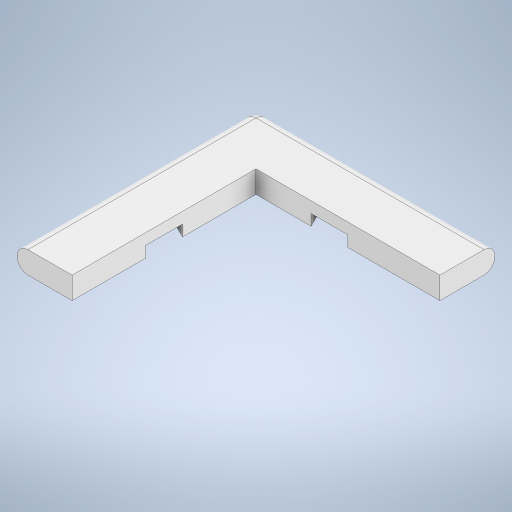
# Autodesk Inventor part: Test2
Saved by Autodesk Inventor 2023.1 (Build 271208000, 208)
## iProperties
Created: 2023-02-07
Part Number: Test2
Material: ABS Plastic
Document SubType Name: Modeling
Designer: 19644
Density: 1.06 g/cm^3
Appearance: Smooth - White
Author: 19644
## iProperties of the stored document Test2_3DPrint.ipt
Created: 2023-02-07
Part Number: Test2_3DPrint
Material: Generic
Document SubType Name: Modeling
Designer: 19644
Density: 1 g/cm^3
Appearance: Default
Author: 19644
Autodesk Inventor part; units mm, degrees
ref_plane "YZ Plane" through (0, 0, 0) normal (1, 0, 0) x (0, 1, 0)
ref_plane "XZ Plane" through (0, 0, 0) normal (0, 1, 0) x (-1, 0, 0)
ref_plane "XY Plane" through (0, 0, 0) normal (0, 0, 1) x (1, 0, 0)
sketch "Sketch1" plane through (0, 0, 0) normal (0, 1, 0) x (-1, 0, 0)
  line L0 (100, -50) -> (-100, -50)
  line L1 (-100, -50) -> (-100, 50)
  line L2 (100, -50) -> (-100, 50) construction
  line L3 (-100, -50) -> (100, 50) construction
  line L4 (-40, -30) -> (-80, -30)
  line L5 (-50, -50) -> (-70, -50)
  line L6 (-40, -30) -> (-50, -50)
  line L7 (-80, -30) -> (-70, -50)
  line L8 (70, -50) -> (50, -50)
  line L9 (-100, -10) -> (-100, 10)
  line L10 (-80, -20) -> (-80, 20)
  line L11 (-80, -20) -> (-100, -10)
  line L12 (-80, 20) -> (-100, 10)
  line L13 (-100, -50) -> (-130, -50)
  line L14 (-130, -50) -> (-130, 50)
  line L15 (-130, 50) -> (-100, 50)
  line L16 (-100, 50) -> (-100, -50)
  line L17 (-130, -50) -> (0, -50)
  line L18 (0, -50) -> (0, -80)
  line L19 (0, -80) -> (-130, -80)
  line L20 (-130, -80) -> (-130, -50)
  line L21 (-40, -70) -> (-80, -70)
  line L22 (-40, -70) -> (-50, -50)
  line L23 (-80, -70) -> (-70, -50)
  line L24 (-120, -20) -> (-120, 20)
  line L25 (-120, -20) -> (-100, -10)
  line L26 (-120, 20) -> (-100, 10)
  line L27 (40, -70) -> (50, -50)
  line L28 (40, -70) -> (80, -70)
  line L29 (80, -70) -> (70, -50)
  line L30 (100, -50) -> (100, 50)
  line L31 (130, -50) -> (130, 50)
  line L32 (130, 50) -> (100, 50)
  line L33 (130, -50) -> (0, -50)
  line L34 (0, -80) -> (130, -80)
  line L35 (130, -80) -> (130, -50)
  line L36 (40, -70) -> (50, -50)
  line L37 (40, -70) -> (80, -70)
  line L38 (80, -70) -> (70, -50)
  line L39 (120, -20) -> (100, -10)
  line L40 (120, 20) -> (100, 10)
  line L41 (120, -20) -> (120, 20)
  point P0 (0, 0)
  point P1 (-100, 10)
  point P2 (-100, -10)
  point P3 (-70, -50)
  point P4 (-50, -50)
  point P5 (0, 0)
  point P6 (0, 0)
  point P7 (0, -50)
  dimension "d72" = 200
  dimension "d73" = 100
  dimension "d78" = 20
  dimension "d79" = 40
  dimension "d80" = 20
  dimension "d81" = 10
  dimension "d82" = 20
  dimension "d86" = 120
  dimension "d88" = 0
  dimension "d90" = 40
  dimension "d91" = 20
  dimension "d92" = 20
  dimension "d93" = 10
  dimension "d94" = 40
  dimension "d95" = 0
  dimension "d114" = 30
  dimension "d115" = 130
  dimension "d116" = 30
  constraints: 84 end point, 15 symmetric about line, 6 horizontal, 4 parallel, 3 midpoint, 3 perpendicular, 2 vertical, 1 coincident
  measures "d72" distance of L1.end L3.end
  measures "d73" distance of L0.end L1.end
  measures "d78" distance of L5.start L5.end
  measures "d79" distance of L4.start L4.end
  measures "d80" distance from line of L5.end L4
  measures "d81" horizontal distance of L4.end L5.end
  measures "d82" distance of L8.start L8.end
  measures "d86" distance of L5.end L8.end
  measures "d88" distance between parallel lines of L0 L5
  measures "d90" distance of L10.start L10.end
  measures "d91" distance of L9.start L9.end
  measures "d92" distance between parallel lines of L9 L10
  measures "d93" vertical distance of L10.start L9.start
  measures "d94" distance from line of L0 L9.start
  measures "d95" distance between parallel lines of L1 L9
  measures "d114" distance of L14.end L15.end
  measures "d115" distance of L18.end L19.end
  measures "d116" distance of L17.end L18.end
extrude "Extrusion24" add sketch "Sketch1" along normal blind 12 contours L33 L35 L34 L18 L0 L27 L28 L29 | L30 L39 L41 L40 L32 L31 L33 | L29 L28 L27 L0 | L30 L40 L41 L39
extrude "Extrusion25" cut sketch "Sketch1" along normal blind 6 contours L29 L28 L27 L0 | L30 L40 L41 L39
fillet "Fillet12" radius 2 4 edges at (-40, 3, -70) (-80, 3, -70) (-120, 3, -20) (-120, 3, 20)
fillet "Fillet13" radius 6 5 edges at (-65, 12, -80) (-65, 0, -80) (-130, 12, -15) (-130, 0, -15) (-130, 6, -80)
body "Solid10"
